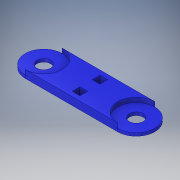
# Autodesk Inventor part: Middle_leg_a
Saved by Autodesk Inventor 2017 (Build 210142000, 142)
## iProperties
Created: 2016-06-08
Part Number: Middle_leg_a
Material: Generic
Document SubType Name: Modeling
Designer: alex-
Density: 1 g/cm^3
Appearance: Blue - Wall Paint - Glossy
Author: alex-
Autodesk Inventor part; units mm, degrees
ref_plane "YZ Plane" through (0, 0, 0) normal (1, 0, 0) x (0, 1, 0)
ref_plane "XZ Plane" through (0, 0, 0) normal (0, 1, 0) x (-1, 0, 0)
ref_plane "XY Plane" through (0, 0, 0) normal (0, 0, 1) x (1, 0, 0)
sketch "Sketch1" plane through (0, 0, 0) normal (0, 1, 0) x (-1, 0, 0)
  circle A0 centre (30, 0) radius 12
  circle A1 centre (-30, 0) radius 12
  line L0 (30, 12) -> (-30, 12)
  line L1 (30, -12) -> (-30, -12)
  circle A2 centre (30, 0) radius 4.5
  circle A3 centre (-30, 0) radius 4.5
  line L2 (58.8, 0) -> (-58.8, 0) projected
  line L3 (2.5, -9) -> (-2.5, -9)
  line L4 (-2.5, -9) -> (-2.5, -4)
  line L5 (-2.5, -4) -> (2.5, -4)
  line L6 (2.5, -4) -> (2.5, -9)
  line L7 (2.5, 9) -> (-2.5, 9)
  line L8 (-2.5, 9) -> (-2.5, 4)
  line L9 (-2.5, 4) -> (2.5, 4)
  line L10 (2.5, 4) -> (2.5, 9)
  point P0 (0, 0)
  point P1 (0, 12)
  point P2 (0, -9)
  point P3 (0, 9)
  dimension "d5" = 60
  dimension "d6" = 24
  dimension "d7" = 9
  dimension "d12" = 5
  dimension "d13" = 5
  dimension "d14" = 4
  constraints: 20 end point, 5 symmetric about line, 4 centre point, 4 point on circle, 3 parallel, 2 coincident, 2 equal radius, 2 horizontal, 2 horizontal alignment, 2 midpoint, 2 tangent, 2 vertical alignment, 1 perpendicular
  measures "d5" distance of A1.centre A0.centre
  measures "d6" diameter of A0
  measures "d7" diameter of A2
  measures "d12" distance of L5.end L3.start
  measures "d13" distance of L3.start L3.end
  measures "d14" distance between parallel lines of L2 L5
extrude "Extrusion2" add sketch "Sketch1" along normal blind 2 contours L2 A2 A0 | A0 L2 A2 | A1 L2 A3 | A1 L2 A3
extrude "Extrusion3" add sketch "Sketch1" along normal blind 5 contours A0 L2 A1 L0 | L1 A1 L2 A0 | L3 L4 L5 L6 | L10 L9 L8 L7
extrude "Extrusion4" cut sketch "Sketch1" along normal up to next contours L3 L4 L5 L6 | L10 L9 L8 L7
equation "\"d6\" = sa_diameter"
equation "\"d7\" = s_shaft_dia"
equation "\"d12\" = b_mat_thickness"
equation "\"d13\" = b_mat_thickness"
equation "\"d14\" = 0.8 * b_mat_thickness"
equation "\"d10\" = b_mat_thickness"
equation "\"sa_diameter\" = 24"
equation "\"s_shaft_dia\" = 9"
equation "\"b_mat_thickness\" = 5"
body "Solid2"
